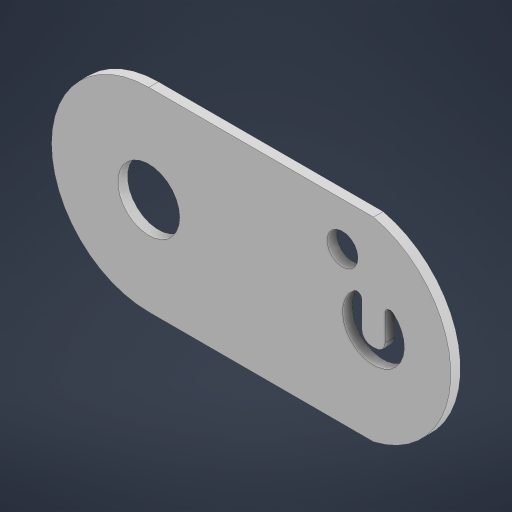
# Autodesk Inventor part: new_winch_pto_poly
Saved by Autodesk Inventor 2023 (Build 270158000, 158)
## iProperties
Created: 2024-04-03
Part Number: new_winch_pto_poly
Material: Generic
Document SubType Name: Modeling
Designer: Meer
Density: 1 g/cm^3
Appearance: Default
Author: Meer
Autodesk Inventor part; units mm, degrees
ref_plane "YZ Plane" through (0, 0, 0) normal (1, 0, 0) x (0, 1, 0)
ref_plane "XZ Plane" through (0, 0, 0) normal (0, 1, 0) x (-1, 0, 0)
ref_plane "XY Plane" through (0, 0, 0) normal (0, 0, 1) x (1, 0, 0)
sketch "Sketch1" plane through (0, 0, 0) normal (0, 0, 1) x (1, 0, 0)
  circle A0 centre (0, 0) radius 15.9766
  line L0 (0, 0) -> (36.9062, 0)
  circle A1 centre (36.9062, 0) radius 15.9766
  line L1 (36.9062, 0) -> (49.6062, 0)
  line L2 (36.9062, 0) -> (36.9062, 15.9766)
  line L3 (36.9062, 0) -> (36.9062, -15.9766)
  arc A2 (36.9062, -15.9766) -> (36.9062, 15.9766) centre (33.2069, 0) ccw
  circle A3 centre (36.9062, 0) radius 5.08
  circle A4 centre (0, 0) radius 5.08
  line L4 (0, 15.9766) -> (36.9062, 15.9766)
  line L5 (36.9062, -15.9766) -> (0, -15.9766)
  line L6 (31.8262, 0) -> (31.8262, 5.08)
  line L7 (31.8262, 5.08) -> (35.0012, 5.08)
  line L8 (35.0012, 5.08) -> (38.8112, 5.08)
  line L9 (38.8112, 5.08) -> (38.8112, -2.54)
  line L10 (38.8112, -2.54) -> (35.0012, -2.54)
  line L11 (35.0012, -2.54) -> (35.0012, 5.08)
  line L12 (36.9062, 5.08) -> (31.8262, 8.89)
  circle A5 centre (31.8262, 8.89) radius 2.54
  point P0 (35.0012, 4.7093)
  point P1 (38.8112, 4.7093)
  dimension "d3" = 10.16
  dimension "d0" = 31.9532
  dimension "d1" = 36.9062
  dimension "d2" = 12.7
  dimension "d4" = 10.16
  dimension "d5" = 3.175
  dimension "d6" = 3.81
  dimension "d7" = 7.62
  dimension "d12" = 6.35
  dimension "d13" = 5.08
  constraints: 26 end point, 9 point on circle, 5 centre point, 5 coincident, 3 horizontal, 3 parallel, 2 perpendicular, 2 point on line, 2 tangent, 1 midpoint, 1 vertical, 3 other
  measures "d0" diameter of A0
  measures "d1" distance of L0.start L0.end
  measures "d2" distance of L1.start L1.end
  measures "d4" diameter of A4
  measures "d5" distance of L6.end L7.end
  measures "d6" distance of L9.end L10.end
  measures "d7" distance of L8.end L9.end
  measures "d12" distance of L12.start L12.end
  measures "d13" diameter of A5
extrude "Extrusion1" add sketch "Sketch1" along normal blind 1.5875 contours A0 | L0 A1 L5 A0 | A0 L4 A1 L0 | A1 L2 L8 L7 L6 L0 | L0 A3 L3 A1 | A2 L1 A3 L9 L8 L2 | L3 A3 L1 A2 | L6 L7 L11 A3 | A3 L9 L1 L2 | L8 L9 A3 | L2 L0 L11 A3 | A3 L11 L8 | L0 L3 L10 L11 | L1 L9 L10 L3
fillet "Fillet1" radius 1.5875 2 edges at (38.8112, -2.54, 0.7937) (35.0012, -2.54, 0.7937)
fillet "Fillet2" radius 0.7937 2 edges at (35.0012, 4.7093, 0.7937) (38.8112, 4.7093, 0.7937)
body "Solid1"
